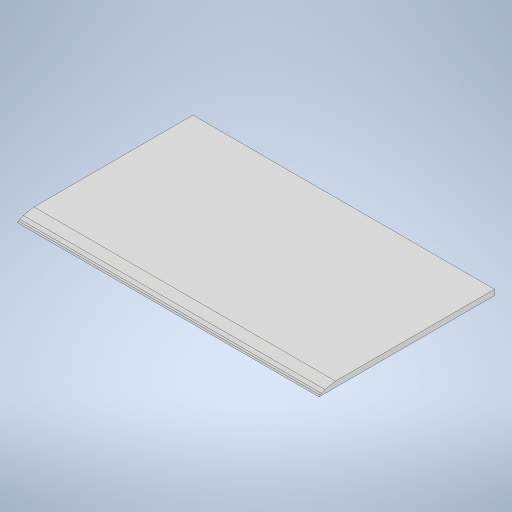
# Autodesk Inventor part: Empuja
Saved by Autodesk Inventor 2024 (Build 280153000, 153)
## iProperties
Created: 2024-04-23
Part Number: Empuja
Material: Generic
Document SubType Name: Modeling
Designer: samue
Density: 1 g/cm^3
Appearance: Default
Author: samue
Autodesk Inventor part; units mm, degrees
ref_plane "YZ Plane" through (0, 0, 0) normal (1, 0, 0) x (0, 1, 0)
ref_plane "XZ Plane" through (0, 0, 0) normal (0, 1, 0) x (-1, 0, 0)
ref_plane "XY Plane" through (0, 0, 0) normal (0, 0, 1) x (1, 0, 0)
sketch "Sketch1" plane through (0, 0, 0) normal (0, 1, 0) x (-1, 0, 0)
  line L0 (55, 25) -> (-55, 25)
  line L1 (-55, 25) -> (-55, -25)
  line L2 (-55, -25) -> (55, -25)
  line L3 (55, -25) -> (55, 25)
  line L4 (55, 25) -> (-55, -25) construction
  line L5 (-55, 25) -> (55, -25) construction
  point P0 (0, 0)
  dimension "d0" = 110
  dimension "d1" = 50
  constraints: 12 end point, 2 midpoint, 2 parallel, 1 horizontal, 1 perpendicular
  measures "d0" distance of L2.end L1.end
  measures "d1" distance of L0.end L1.end
extrude "Extrusion1" add sketch "Sketch1" along normal blind 2
sketch "Sketch2" plane through (55, 0, -25) normal (0, 0, -1) x (-1, 0, 0)
  line L0 (0, 2) -> (110, 2) projected
  line L1 (110, 0.5858) -> (110, 0) projected
  line L2 (0, 2) -> (110, 2)
  line L3 (110, 2) -> (110, 0)
  line L4 (110, 0) -> (0, 0)
  line L5 (0, 0) -> (0, 2)
  point P0 (55, 0)
  constraints: 8 end point, 2 parallel, 1 horizontal, 1 perpendicular
extrude "Extrusion2" add sketch "Sketch2" along normal blind 14
chamfer "Chamfer4" distance 2 angle 45 1 edges at (0, 2, 25)
chamfer "Chamfer5" distance 2 angle 45 1 edges at (0, 2, 23.0001)
chamfer "Chamfer6" distance 2 angle 45 1 edges at (0, 2, 21.0001)
chamfer "Chamfer7" distance 0.3 angle 45 1 edges at (0, 0.5858, 24.4143)
body "Solid1"
